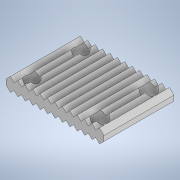
# Autodesk Inventor part: g2Tensioner
Saved by Autodesk Inventor 2020 (Build 240168000, 168)
## iProperties
Created: 2021-06-02
Part Number: g2Tensioner
Material: Generic
Document SubType Name: Modeling
Designer: PAB
Density: 1 g/cm^3
Appearance: Default
Author: PAB
Autodesk Inventor part; units mm, degrees
ref_plane "YZ Plane" through (0, 0, 0) normal (1, 0, 0) x (0, 1, 0)
ref_plane "XZ Plane" through (0, 0, 0) normal (0, 1, 0) x (-1, 0, 0)
ref_plane "XY Plane" through (0, 0, 0) normal (0, 0, 1) x (1, 0, 0)
sketch "Sketch1" plane through (0, 0, 0) normal (0, 1, 0) x (-1, 0, 0)
  line L0 (14, 12) -> (-14, 12)
  line L1 (-14, 12) -> (-14, -8)
  line L2 (-14, -8) -> (14, -8)
  line L3 (14, -8) -> (14, 12)
  point P0 (0, 0)
  dimension "d0" = 28
  dimension "d1" = 20
  dimension "d4" = 14
  constraints: 8 end point, 2 parallel, 1 horizontal, 1 perpendicular
  measures "d0" distance of L2.end L1.end
  measures "d1" distance of L1.end L0.end
  measures "d4" distance from line of point (0, 0) L1
extrude "Extrusion1" add sketch "Sketch1" along normal mid plane 4
sketch "Sketch2" plane through (-14, 2, 12) normal (0, 0, 1) x (1, 0, 0)
  line L0 (0, 0) -> (28, 0) projected
  line L1 (14, 0) -> (12.9393, -1.0607)
  line L2 (14, 0) -> (15.5, 0) construction
  line L3 (12.9393, -1.0607) -> (11.8787, 0)
  line L4 (11.8787, 0) -> (10.818, -1.0607)
  line L5 (10.818, -1.0607) -> (9.7574, 0)
  line L6 (9.7574, 0) -> (8.6967, -1.0607)
  line L7 (8.6967, -1.0607) -> (7.636, 0)
  line L8 (7.636, 0) -> (6.5754, -1.0607)
  line L9 (6.5754, -1.0607) -> (5.5147, 0)
  line L10 (5.5147, 0) -> (4.4541, -1.0607)
  line L11 (4.4541, -1.0607) -> (3.3934, 0)
  line L12 (3.3934, 0) -> (2.3327, -1.0607)
  line L13 (2.3327, -1.0607) -> (1.2721, 0)
  line L14 (1.2721, 0) -> (0, -1.2721)
  line L15 (0, -4) -> (0, 0) projected
  line L16 (14, 0) -> (15.0607, -1.0607)
  line L17 (15.0607, -1.0607) -> (16.1213, 0)
  line L18 (16.1213, 0) -> (17.182, -1.0607)
  line L19 (17.182, -1.0607) -> (18.2426, 0)
  line L20 (18.2426, 0) -> (19.3033, -1.0607)
  line L21 (19.3033, -1.0607) -> (20.364, 0)
  line L22 (20.364, 0) -> (21.4246, -1.0607)
  line L23 (21.4246, -1.0607) -> (22.4853, 0)
  line L24 (22.4853, 0) -> (23.5459, -1.0607)
  line L25 (23.5459, -1.0607) -> (24.6066, 0)
  line L26 (24.6066, 0) -> (25.6673, -1.0607)
  line L27 (25.6673, -1.0607) -> (26.7279, 0)
  line L28 (26.7279, 0) -> (28, -1.2721)
  line L29 (28, -4) -> (28, 0) projected
  point P0 (14, -2)
  point P1 (1.2721, 0)
  point P2 (1.2721, 0)
  point P3 (5.5147, 0)
  point P4 (5.5147, 0)
  point P5 (7.636, 0)
  point P6 (7.636, 0)
  point P7 (9.7574, 0)
  point P8 (9.7574, 0)
  dimension "d5" = 1.5
  dimension "d6" = 135
  dimension "d7" = 1.5
  constraints: 54 end point, 25 perpendicular, 2 point on line, 1 equal length, 1 horizontal, 3 other
  measures "d5" distance of L1.start L1.end
  measures "d6" angle of L1 L2
  measures "d7" distance of L3.end L4.end
extrude "Extrusion2" cut sketch "Sketch2" against normal blind 50
mirror "Mirror1" about plane through (0, 0, 0) normal (0, 1, 0) of "Extrusion2"
sketch "Sketch4" plane through (0, 0, 0) normal (0, 1, 0) x (-1, 0, 0)
  circle A0 centre (9.757, -5) radius 2
  circle A1 centre (-9.757, -5) radius 2
  circle A2 centre (-9.757, 9) radius 2
  circle A3 centre (9.757, 9) radius 2
  point P0 (0, 0)
  dimension "d14" = 4
  dimension "d15" = 4
  dimension "d16" = 4
  dimension "d17" = 4
  constraints: 4 centre point
  measures "d14" diameter of A0
  measures "d15" diameter of A1
  measures "d16" diameter of A2
  measures "d17" diameter of A3
extrude "Extrusion4" cut sketch "Sketch4" against normal mid plane 6
body "Solid1"
